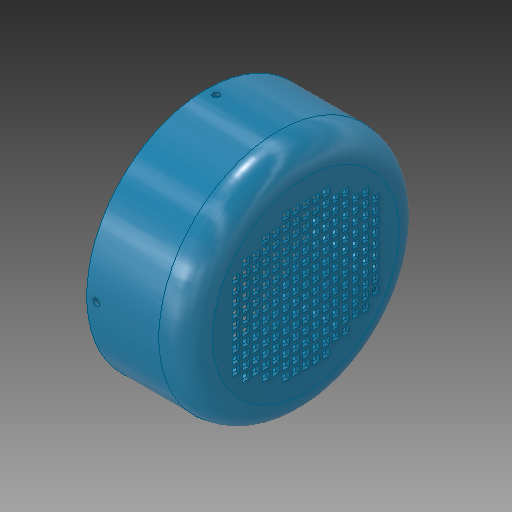
# Autodesk Inventor part: nap sau
Saved by Autodesk Inventor 2019 (Build 230136000, 136)
## iProperties
Created: 2017-11-11
Part Number: nap sau
Material: Stainless Steel
Document SubType Name: Modeling
Designer: Mr.Duc
Density: 8 g/cm^3
Appearance: Sky Blue Dark
Author: Mr.Duc
Autodesk Inventor part; units mm, degrees
ref_plane "YZ Plane" through (0, 0, 0) normal (1, 0, 0) x (0, 1, 0)
ref_plane "XZ Plane" through (0, 0, 0) normal (0, 1, 0) x (-1, 0, 0)
ref_plane "XY Plane" through (0, 0, 0) normal (0, 0, 1) x (1, 0, 0)
sketch "Sketch1" plane through (0, 0, 0) normal (0, 0, 1) x (1, 0, 0)
  line L0 (0, 0) -> (0, 174.8352) construction
  line L1 (-105.6274, 175) -> (-105.6274, 180)
  line L2 (-105.6274, 180) -> (2.9584, 180)
  arc A0 (44.3726, 140.5078) -> (2.9584, 180) centre (2.9584, 138.539) ccw
  line L3 (44.3726, 140.5078) -> (44.3726, 0)
  line L4 (-132.9998, 0) -> (225.6473, 0) construction
  line L5 (39.3726, 0) -> (39.3726, 136.6927)
  arc A1 (39.3726, 136.6927) -> (2.9584, 175) centre (2.9584, 138.539) ccw
  line L6 (2.9584, 175) -> (-100.6274, 175)
  line L7 (39.3726, 0) -> (44.3726, 0)
  line L8 (-105.6274, 175) -> (-100.6274, 175)
  line L9 (0, 0) -> (39.3726, 0)
  dimension "d2" = 150
  dimension "d3" = 5
  dimension "d5" = 175
  dimension "d6" = 5
  constraints: 20 end point, 4 horizontal, 4 point on circle, 3 collinear, 2 centre point, 2 vertical, 1 coincident, 1 perpendicular, 1 point on line, 1 tangent, 4 other
  measures "d2" distance from line of L1.end L3
  measures "d3" distance between parallel lines of L3 L5
  measures "d5" distance between parallel lines of L9 L6
  measures "d6" distance between parallel lines of L6 L2
revolve "Revolution1" add sketch "Sketch1" angle 360 about axis through (0, 0, 0) along (1, 0, 0)
sketch "Sketch2" plane through (44.3726, 0, 0) normal (1, 0, 0) x (0, 0, -1)
  line L0 (0, 0) -> (0, -195) construction
  line L1 (0, 0) -> (0, -145.0216) construction
  line L2 (0, 0) -> (-156, 0) construction
  line L3 (5, -5) -> (-5, -5)
  line L4 (-5, -5) -> (-5, 5)
  line L5 (-5, 5) -> (5, 5)
  line L6 (5, 5) -> (5, -5)
  line L7 (5, -5) -> (-5, 5) construction
  line L8 (-5, -5) -> (5, 5) construction
  dimension "d7" = 10
  dimension "d8" = 10
  constraints: 18 end point, 2 horizontal, 2 midpoint, 2 parallel, 2 vertical, 1 perpendicular
  measures "d7" distance of L4.end L5.end
  measures "d8" distance of L5.end L3.start
extrude "Extrusion1" cut sketch "Sketch2" against normal blind 52.75
pattern_linear "Rectangular Pattern1" count 8 spacing 15 along (0, -1, 0) of "Extrusion1"
pattern_linear "Rectangular Pattern2" count 8 spacing 15 along (0, 1, 0) of "Extrusion1"
pattern_linear "Rectangular Pattern3" count 3 spacing 15 along (0, 0, 1) count 3 spacing 15 along (0, 0, -1) of "Extrusion1", "Rectangular Pattern2", "Rectangular Pattern1"
sketch "Sketch3" plane through (44.3726, 0, 0) normal (1, 0, 0) x (0, 0, -1)
  line L0 (-50, -5) -> (-40, -5)
  line L1 (-40, -5) -> (-40, 5)
  line L2 (-40, 5) -> (-50, 5)
  line L3 (-50, 5) -> (-50, -5)
  line L4 (-50, -5) -> (-40, 5) construction
  line L5 (-40, -5) -> (-50, 5) construction
  line L6 (-35, -5) -> (-35, 5) projected
  line L7 (-35, 5) -> (-25, 5) projected
  point P0 (0, 0)
  point P1 (-45, 0)
  dimension "d23" = 10
  dimension "d24" = 10
  dimension "d26" = 5
  constraints: 12 end point, 2 midpoint, 2 parallel, 1 collinear, 1 horizontal, 1 perpendicular
  measures "d23" distance of L0.start L0.end
  measures "d24" distance of L0.end L1.end
  measures "d26" distance between parallel lines of L6 L1
extrude "Extrusion2" cut sketch "Sketch3" against normal blind 52.75
pattern_linear "Rectangular Pattern4" count 7 spacing 15 along (0, -1, 0) count 7 spacing 15 along (0, 1, 0) of "Extrusion2"
pattern_linear "Rectangular Pattern5" count 2 spacing 15 along (0, 0, 1) of "Extrusion2", "Rectangular Pattern4"
sketch "Sketch4" plane through (44.3726, 0, 0) normal (1, 0, 0) x (0, 0, -1)
  line L0 (-80, -5) -> (-70, -5)
  line L1 (-70, -5) -> (-70, 5)
  line L2 (-70, 5) -> (-80, 5)
  line L3 (-80, 5) -> (-80, -5)
  line L4 (-80, -5) -> (-70, 5) construction
  line L5 (-70, -5) -> (-80, 5) construction
  line L6 (-65, -5) -> (-65, 5) projected
  line L7 (-65, 5) -> (-55, 5) projected
  point P0 (0, 0)
  point P1 (-75, 0)
  dimension "d38" = 10
  dimension "d39" = 10
  dimension "d40" = 5
  constraints: 12 end point, 2 midpoint, 2 parallel, 1 collinear, 1 horizontal, 1 perpendicular
  measures "d38" distance of L1.end L2.end
  measures "d39" distance of L0.end L1.end
  measures "d40" distance between parallel lines of L6 L1
extrude "Extrusion3" cut sketch "Sketch4" against normal blind 52.75
pattern_linear "Rectangular Pattern6" count 6 spacing 15 along (0, -1, 0) count 6 spacing 15 along (0, 1, 0) of "Extrusion3"
pattern_linear "Rectangular Pattern7" count 2 spacing 15 along (0, 0, 1) of "Extrusion3", "Rectangular Pattern6"
mirror "Mirror1" about plane through (0, 0, 0) normal (0, 0, 1) of "Extrusion3", "Rectangular Pattern6", "Rectangular Pattern7", "Extrusion2", "Rectangular Pattern4", "Rectangular Pattern5"
sketch "Sketch6" plane through (44.3726, 0, 0) normal (1, 0, 0) x (0, 0, -1)
  line L0 (-110, -5) -> (-100, -5)
  line L1 (-100, -5) -> (-100, 5)
  line L2 (-100, 5) -> (-110, 5)
  line L3 (-110, 5) -> (-110, -5)
  line L4 (-110, -5) -> (-100, 5) construction
  line L5 (-100, -5) -> (-110, 5) construction
  line L6 (-95, -5) -> (-95, 5) projected
  line L7 (-95, 5) -> (-85, 5) projected
  line L8 (-110, -20) -> (-100, -20)
  line L9 (-100, -20) -> (-100, -10)
  line L10 (-100, -10) -> (-110, -10)
  line L11 (-110, -10) -> (-110, -20)
  line L12 (-110, -20) -> (-100, -10) construction
  line L13 (-100, -20) -> (-110, -10) construction
  line L14 (-110, -35) -> (-100, -35)
  line L15 (-100, -35) -> (-100, -25)
  line L16 (-100, -25) -> (-110, -25)
  line L17 (-110, -25) -> (-110, -35)
  line L18 (-110, -35) -> (-100, -25) construction
  line L19 (-100, -35) -> (-110, -25) construction
  line L20 (-110, -50) -> (-100, -50)
  line L21 (-100, -50) -> (-100, -40)
  line L22 (-100, -40) -> (-110, -40)
  line L23 (-110, -40) -> (-110, -50)
  line L24 (-110, -50) -> (-100, -40) construction
  line L25 (-100, -50) -> (-110, -40) construction
  line L26 (-110, -65) -> (-100, -65)
  line L27 (-100, -65) -> (-100, -55)
  line L28 (-100, -55) -> (-110, -55)
  line L29 (-110, -55) -> (-110, -65)
  line L30 (-110, -65) -> (-100, -55) construction
  line L31 (-100, -65) -> (-110, -55) construction
  line L32 (-110, 10) -> (-100, 10)
  line L33 (-100, 10) -> (-100, 20)
  line L34 (-100, 20) -> (-110, 20)
  line L35 (-110, 20) -> (-110, 10)
  line L36 (-110, 10) -> (-100, 20) construction
  line L37 (-100, 10) -> (-110, 20) construction
  line L38 (-110, -5) -> (-100, -5)
  line L39 (-100, -5) -> (-100, 5)
  line L40 (-100, 5) -> (-110, 5)
  line L41 (-110, 5) -> (-110, -5)
  line L42 (-110, -5) -> (-100, 5) construction
  line L43 (-100, -5) -> (-110, 5) construction
  line L44 (-110, -20) -> (-100, -20)
  line L45 (-100, -20) -> (-100, -10)
  line L46 (-100, -10) -> (-110, -10)
  line L47 (-110, -10) -> (-110, -20)
  line L48 (-110, -20) -> (-100, -10) construction
  line L49 (-100, -20) -> (-110, -10) construction
  line L50 (-110, -35) -> (-100, -35)
  line L51 (-100, -35) -> (-100, -25)
  line L52 (-100, -25) -> (-110, -25)
  line L53 (-110, -25) -> (-110, -35)
  line L54 (-110, -35) -> (-100, -25) construction
  line L55 (-100, -35) -> (-110, -25) construction
  line L56 (-110, -50) -> (-100, -50)
  line L57 (-100, -50) -> (-100, -40)
  line L58 (-100, -40) -> (-110, -40)
  line L59 (-110, -40) -> (-110, -50)
  line L60 (-110, -50) -> (-100, -40) construction
  line L61 (-100, -50) -> (-110, -40) construction
  line L62 (-110, 25) -> (-100, 25)
  line L63 (-100, 25) -> (-100, 35)
  line L64 (-100, 35) -> (-110, 35)
  line L65 (-110, 35) -> (-110, 25)
  line L66 (-110, 25) -> (-100, 35) construction
  line L67 (-100, 25) -> (-110, 35) construction
  line L68 (-110, 10) -> (-100, 10)
  line L69 (-100, 10) -> (-100, 20)
  line L70 (-100, 20) -> (-110, 20)
  line L71 (-110, 20) -> (-110, 10)
  line L72 (-110, 10) -> (-100, 20) construction
  line L73 (-100, 10) -> (-110, 20) construction
  line L74 (-110, -5) -> (-100, -5)
  line L75 (-100, -5) -> (-100, 5)
  line L76 (-100, 5) -> (-110, 5)
  line L77 (-110, 5) -> (-110, -5)
  line L78 (-110, -5) -> (-100, 5) construction
  line L79 (-100, -5) -> (-110, 5) construction
  line L80 (-110, -20) -> (-100, -20)
  line L81 (-100, -20) -> (-100, -10)
  line L82 (-100, -10) -> (-110, -10)
  line L83 (-110, -10) -> (-110, -20)
  line L84 (-110, -20) -> (-100, -10) construction
  line L85 (-100, -20) -> (-110, -10) construction
  line L86 (-110, -35) -> (-100, -35)
  line L87 (-100, -35) -> (-100, -25)
  line L88 (-100, -25) -> (-110, -25)
  line L89 (-110, -25) -> (-110, -35)
  line L90 (-110, -35) -> (-100, -25) construction
  line L91 (-100, -35) -> (-110, -25) construction
  line L92 (-110, 40) -> (-100, 40)
  line L93 (-100, 40) -> (-100, 50)
  line L94 (-100, 50) -> (-110, 50)
  line L95 (-110, 50) -> (-110, 40)
  line L96 (-110, 40) -> (-100, 50) construction
  line L97 (-100, 40) -> (-110, 50) construction
  line L98 (-110, 25) -> (-100, 25)
  line L99 (-100, 25) -> (-100, 35)
  line L100 (-100, 35) -> (-110, 35)
  line L101 (-110, 35) -> (-110, 25)
  line L102 (-110, 25) -> (-100, 35) construction
  line L103 (-100, 25) -> (-110, 35) construction
  line L104 (-110, 10) -> (-100, 10)
  line L105 (-100, 10) -> (-100, 20)
  line L106 (-100, 20) -> (-110, 20)
  line L107 (-110, 20) -> (-110, 10)
  line L108 (-110, 10) -> (-100, 20) construction
  line L109 (-100, 10) -> (-110, 20) construction
  line L110 (-110, -5) -> (-100, -5)
  line L111 (-100, -5) -> (-100, 5)
  line L112 (-100, 5) -> (-110, 5)
  line L113 (-110, 5) -> (-110, -5)
  line L114 (-110, -5) -> (-100, 5) construction
  line L115 (-100, -5) -> (-110, 5) construction
  line L116 (-110, -20) -> (-100, -20)
  line L117 (-100, -20) -> (-100, -10)
  line L118 (-100, -10) -> (-110, -10)
  line L119 (-110, -10) -> (-110, -20)
  line L120 (-110, -20) -> (-100, -10) construction
  line L121 (-100, -20) -> (-110, -10) construction
  line L122 (-110, 55) -> (-100, 55)
  line L123 (-100, 55) -> (-100, 65)
  line L124 (-100, 65) -> (-110, 65)
  line L125 (-110, 65) -> (-110, 55)
  line L126 (-110, 55) -> (-100, 65) construction
  line L127 (-100, 55) -> (-110, 65) construction
  line L128 (-110, 40) -> (-100, 40)
  line L129 (-100, 40) -> (-100, 50)
  line L130 (-100, 50) -> (-110, 50)
  line L131 (-110, 50) -> (-110, 40)
  line L132 (-110, 40) -> (-100, 50) construction
  line L133 (-100, 40) -> (-110, 50) construction
  line L134 (-110, 25) -> (-100, 25)
  line L135 (-100, 25) -> (-100, 35)
  line L136 (-100, 35) -> (-110, 35)
  line L137 (-110, 35) -> (-110, 25)
  line L138 (-110, 25) -> (-100, 35) construction
  line L139 (-100, 25) -> (-110, 35) construction
  line L140 (-110, 10) -> (-100, 10)
  line L141 (-100, 10) -> (-100, 20)
  line L142 (-100, 20) -> (-110, 20)
  line L143 (-110, 20) -> (-110, 10)
  line L144 (-110, 10) -> (-100, 20) construction
  line L145 (-100, 10) -> (-110, 20) construction
  line L146 (-110, -5) -> (-100, -5)
  line L147 (-100, -5) -> (-100, 5)
  line L148 (-100, 5) -> (-110, 5)
  line L149 (-110, 5) -> (-110, -5)
  line L150 (-110, -5) -> (-100, 5) construction
  line L151 (-100, -5) -> (-110, 5) construction
  point P0 (0, 0)
  point P1 (-105, 0)
  point P2 (-105, -15)
  point P3 (-105, -30)
  point P4 (-105, -45)
  point P5 (-105, -60)
  point P6 (-105, 15)
  point P7 (-105, 0)
  point P8 (-105, -15)
  point P9 (-105, -30)
  point P10 (-105, -45)
  point P11 (-105, 30)
  point P12 (-105, 15)
  point P13 (-105, 0)
  point P14 (-105, -15)
  point P15 (-105, -30)
  point P16 (-105, 45)
  point P17 (-105, 30)
  point P18 (-105, 15)
  point P19 (-105, 0)
  point P20 (-105, -15)
  point P21 (-105, 60)
  point P22 (-105, 45)
  point P23 (-105, 30)
  point P24 (-105, 15)
  point P25 (-105, 0)
  dimension "d52" = 10
  dimension "d53" = 10
  dimension "d54" = 5
  dimension "d57" = 15
  dimension "d60" = 15
  constraints: 300 end point, 50 midpoint, 3 collinear, 2 parallel, 2 vertical, 1 horizontal, 1 perpendicular, 262 other
  measures "d52" distance of L0.start L0.end
  measures "d53" distance of L0.end L1.end
  measures "d54" distance between parallel lines of L6 L1
  measures "d57" distance of L0.start L8.start
  measures "d60" distance of L0.start L32.start
extrude "Extrusion4" cut sketch "Sketch6" against normal blind 52.75
mirror "Mirror2" about plane through (0, 0, 0) normal (0, 0, 1) of "Extrusion4"
sketch "Sketch7" plane through (0, 0, 0) normal (0, 1, 0) x (-1, 0, 0)
  circle A0 centre (90.6274, 0) radius 5
  line L0 (105.6274, 175) -> (105.6274, -175) projected
  point P0 (0, 0)
  dimension "d65" = 10
  dimension "d66" = 15
  constraints: 1 centre point
  measures "d65" diameter of A0
  measures "d66" distance from line of L0 A0.centre
extrude "Extrusion5" cut sketch "Sketch7" along normal through all both and the other way through all
pattern_circular "Circular Pattern1" count 4 over 360 about axis through (-103.1274, 0, 0) along (1, 0, 0) of "Extrusion5"
body "Solid1"
